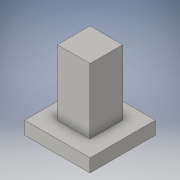
# Autodesk Inventor part: Piece
Saved by Autodesk Inventor 2016 (Build 200138000, 138)
## iProperties
Created: 2015-09-14
Part Number: Piece
Material: Generic
Document SubType Name: Modeling
Designer: Pranav
Density: 1 g/cm^3
Appearance: Default
Author: Pranav
Autodesk Inventor part; units mm, degrees
ref_plane "YZ Plane" through (0, 0, 0) normal (1, 0, 0) x (0, 1, 0)
ref_plane "XZ Plane" through (0, 0, 0) normal (0, 1, 0) x (-1, 0, 0)
ref_plane "XY Plane" through (0, 0, 0) normal (0, 0, 1) x (1, 0, 0)
sketch "Sketch1" plane through (0, 0, 0) normal (0, 1, 0) x (-1, 0, 0)
  line L0 (0, 0) -> (254, 0)
  line L1 (254, 0) -> (254, -254)
  line L2 (254, -254) -> (0, -254)
  line L3 (0, -254) -> (0, 0)
  dimension "d0" = 254
  dimension "d1" = 254
  constraints: 8 end point, 2 parallel, 1 horizontal, 1 perpendicular
  measures "d0" distance of L1.end L2.end
  measures "d1" distance of L0.end L1.end
extrude "Extrusion1" add sketch "Sketch1" along normal blind 50.8
sketch "Sketch2" plane through (0, 50.8, 0) normal (0, 1, 0) x (1, 0, 0)
  line L0 (-190.5, 63.5) -> (-63.5, 63.5)
  line L1 (-63.5, 63.5) -> (-63.5, 190.5)
  line L2 (-63.5, 190.5) -> (-190.5, 190.5)
  line L3 (-190.5, 190.5) -> (-190.5, 63.5)
  point P0 (0, 0)
  dimension "d4" = 127
  dimension "d5" = 127
  dimension "d6" = 63.5
  dimension "d7" = 190.5
  constraints: 8 end point, 2 parallel, 1 horizontal, 1 perpendicular
  measures "d4" distance between parallel lines of L1 L3
  measures "d5" distance between parallel lines of L0 L2
  measures "d6" distance from line of point (0, 0) L1
  measures "d7" distance from line of point (0, 0) L2
extrude "Extrusion2" add sketch "Sketch2" along normal blind 254
body "Solid1"
